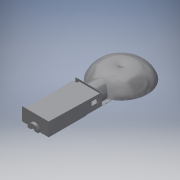
# Autodesk Inventor part: Shelter
Saved by Autodesk Inventor 2017 (Build 210142000, 142)
## iProperties
Created: 2021-04-11
Part Number: Shelter
Material: Aluminum 6061-AHC
Document SubType Name: Modeling
Designer: udays
Density: 2.7 g/cm^3
Appearance: Aluminum Cast
Author: udays
Autodesk Inventor part; units mm, degrees
ref_plane "YZ Plane" through (0, 0, 0) normal (1, 0, 0) x (0, 1, 0)
ref_plane "XZ Plane" through (0, 0, 0) normal (0, 1, 0) x (-1, 0, 0)
ref_plane "XY Plane" through (0, 0, 0) normal (0, 0, 1) x (1, 0, 0)
sketch "Sketch1" plane through (0, 0, 0) normal (0, 1, 0) x (-1, 0, 0)
  line L0 (0, 0) -> (2540, 0)
  line L1 (2540, 0) -> (2540, -5080)
  line L2 (2540, -5080) -> (0, -5080)
  line L3 (0, -5080) -> (0, 0)
  dimension "d0" = 2540
  dimension "d1" = 5080
  constraints: 8 end point, 2 parallel, 1 horizontal, 1 perpendicular
  measures "d0" distance of L1.end L2.end
  measures "d1" distance of L0.end L1.end
extrude "Extrusion1" add sketch "Sketch1" along normal blind 25.4
sketch "Sketch2" plane through (-2540, 0, 0) normal (0, 0, 1) x (1, 0, 0)
  line L0 (2540, 0) -> (0, 0) projected
  line L1 (0, 0) -> (2540, 0)
  line L2 (2540, 0) -> (2540, 1270)
  line L3 (2540, 1270) -> (0, 1270)
  line L4 (0, 1270) -> (0, 0)
  dimension "d4" = 1270
  constraints: 8 end point, 2 parallel, 1 horizontal, 1 perpendicular
  measures "d4" distance of L2.end L1.end
extrude "Extrusion2" add sketch "Sketch2" along normal blind 25.4
sketch "Sketch3" plane through (0, 25.4, 0) normal (1, 0, 0) x (0, 0, -1)
  line L0 (5080, -25.4) -> (-25.4, -25.4) projected
  line L1 (-25.4, -25.4) -> (5105.4, -25.4)
  line L2 (5105.4, -25.4) -> (5105.4, 1117.6)
  line L3 (-25.4, 1244.6) -> (-25.4, -25.4) projected
  line L4 (-25.4, -25.4) -> (-25.4, 1244.6)
  line L5 (-25.4, 1244.6) -> (5105.4, 1117.6)
  point P0 (0, -25.4)
  dimension "d8" = 1143
  dimension "d35" = 1270
  constraints: 8 end point, 1 collinear, 1 horizontal, 1 perpendicular
  measures "d8" distance of L2.end L1.end
  measures "d35" distance of L0.end L3.start
extrude "Extrusion3" add sketch "Sketch3" along normal blind 25.4
sketch "Sketch4" plane through (0, 0, -5105.4) normal (0, 0, -1) x (-1, 0, 0)
  arc A0 (2159, 0) -> (1270, 889) centre (1270, 0) ccw
  arc A1 (1270, 889) -> (381, 0) centre (1270, 0) ccw
  line L0 (2540, 1143) -> (5105.4, 1143) construction
  line L1 (2540, 0) -> (-25.4, 0) projected
  line L2 (2540, 0) -> (2540, 1143)
  line L3 (2540, 1143) -> (-25.4, 1143)
  line L4 (-25.4, 1143) -> (-25.4, 0)
  line L5 (-25.4, 0) -> (381, 0)
  line L6 (2159, 0) -> (2540, 0)
  dimension "d32" = 1143
  constraints: 12 end point, 5 point on circle, 3 horizontal, 3 parallel, 2 centre point, 2 perpendicular, 1 coincident
  measures "d32" distance of L0.start L2.start
ref_plane "Work Plane1" through (0, 0, -5130.8) normal (0, 0, -1) x (-1, 0, 0)
sketch "Sketch7" plane through (0, 0, -5130.8) normal (0, 0, -1) x (-1, 0, 0)
  line L0 (2540, 0) -> (0, 0) projected
  arc A0 (2235.2, 0) -> (1270, 965.2) centre (1270, 0) ccw
  arc A1 (1270, 965.2) -> (304.8, 0) centre (1270, 0) ccw
  line L1 (304.8, 0) -> (2235.2, 0)
  dimension "d17" = 965.2
  constraints: 4 point on circle, 2 centre point, 2 end point, 1 coincident, 1 collinear, 1 midpoint
  measures "d17" radius of A0
extrude "Extrusion6" add sketch "Sketch7" along normal blind 1536.7
extrude "Extrusion9" add sketch "Sketch4" along normal blind 25.4 contours A0 A1 L1 L4 L3 L2
sketch "Sketch12" plane through (0, 0, -5080) normal (0, 0, -1) x (-1, 0, 0)
  line L0 (2540, 0) -> (-25.4, 0) projected
  line L1 (2540, 1270) -> (2540, 25.4) projected
  line L2 (-25.4, 0) -> (2540, 0)
  line L3 (2540, 0) -> (2540, 25.4)
  line L4 (2540, 25.4) -> (-25.4, 25.4)
  line L5 (-25.4, 25.4) -> (-25.4, 0)
  point P0 (0, 0)
  constraints: 8 end point, 2 parallel, 1 horizontal, 1 perpendicular
extrude "Extrusion11" add sketch "Sketch12" along normal blind 1898.65
fillet "Fillet2" radius 39.6875 1 edges at (-1270, 889, -5130.8)
ref_plane "Work Plane4" through (0, 0, -8262.4422) normal (0, 0, -1) x (-1, 0, 0)
sketch "Sketch14" plane through (0, 0, -8262.4422) normal (0, 0, -1) x (-1, 0, 0)
  line L0 (2540, 25.4) -> (0, 25.4) projected
  line L1 (1270, 25.4) -> (3810, 25.4)
  line L2 (1270, 25.4) -> (1270, 1117.6)
  arc A0 (3810, 25.4) -> (1270, 1117.6) centre (2045.9544, -577.4432) ccw
  point P0 (0, 0)
  dimension "d48" = 2540
  dimension "d49" = 1092.2
  constraints: 4 end point, 2 point on circle, 1 centre point, 1 collinear, 1 midpoint, 1 perpendicular
  measures "d48" distance of L1.start L1.end
  measures "d49" distance of L1.start L2.end
revolve "Revolution1" add sketch "Sketch14" angle 360 about axis through (-1270, 25.4, -8262.4422) along (0, 1, 0)
sketch "Sketch16" plane through (0, 0, -5130.8) normal (0, 0, 1) x (1, 0, 0)
  line L0 (25.4, 0) -> (-2540, 0) projected
  line L1 (-1257.3, 0) -> (-1257.3, 28.575)
  arc A0 (-495.3, 28.575) -> (-1257.3, 790.575) centre (-1257.3, 28.575) ccw
  line L2 (-1257.3, 28.575) -> (-1257.3, 790.575) construction
  line L3 (-1257.3, 28.575) -> (-495.3, 28.575) construction
  line L4 (-1257.3, 28.575) -> (-495.3, 28.575) construction
  arc A1 (-1257.3, 790.575) -> (-2019.3, 28.575) centre (-1257.3, 28.575) ccw
  line L5 (-1257.3, 28.575) -> (-2019.3, 28.575) construction
  line L6 (-1257.3, 28.575) -> (-1257.3, 790.575) construction
  arc A2 (-495.3, 28.575) -> (-2019.3, 28.575) centre (-1257.3, 28.575) ccw
  line L7 (-2019.3, 28.575) -> (-495.3, 28.575)
  point P0 (0, 0)
  dimension "d51" = 28.575
  dimension "d52" = 762
  dimension "d53" = 90
  dimension "d54" = 90
  dimension "d55" = 90
  constraints: 14 end point, 7 point on circle, 3 centre point, 2 coincident, 1 concentric, 1 horizontal, 1 midpoint, 1 perpendicular, 1 vertical
  measures "d51" distance of L1.start L1.end
  measures "d52" radius of A0
  measures "d53" angle of L3 L2
  measures "d54" angle of L4 L2
  measures "d55" angle of L6 L5
extrude "Extrusion12" cut sketch "Sketch16" against normal blind 5027.6125
sketch "Sketch18" plane through (-2540, 0, 25.4) normal (0, 0, 1) x (1, 0, 0)
  arc A0 (2121.4941, 28.575) -> (419.2797, 46.1929) centre (1270, 0) ccw projected
  line L0 (1786.8174, 24.4898) -> (770.8174, 24.4898) construction
  line L1 (1786.8174, 24.4898) -> (2802.8174, 24.4898) construction
  line L2 (770.8174, 24.4898) -> (1786.8174, 24.4898)
  arc A1 (1786.8174, 24.4898) -> (770.8174, 24.4898) centre (1278.8174, 49.8239) ccw
  point P0 (2540, 0)
  point P1 (1278.8174, 532.4898)
  dimension "d62" = 1016
  dimension "d63" = 180
  constraints: 6 end point, 2 collinear, 2 point on circle, 1 centre point, 1 horizontal
  measures "d62" distance of L0.start L0.end
  measures "d63" angle of L0 L1
extrude "Extrusion13" add sketch "Sketch18" along normal blind 254
sketch "Sketch19" plane through (0, 25.4, 0) normal (0, 1, 0) x (1, 0, 0)
  line L0 (0, 5105.4) -> (0, 0) projected
  line L1 (0, 0) -> (-2540, 0) projected
  line L2 (0, 1699.357) -> (-752.9015, 1699.357)
  line L3 (-752.9015, 1699.357) -> (-752.9015, 0)
  line L4 (-752.9015, 0) -> (0, 0)
  line L5 (0, 0) -> (0, 1699.357)
  line L6 (0, 0) -> (-726.44, 0)
  line L7 (-726.44, 0) -> (-726.44, 1673.86)
  line L8 (-726.44, 1673.86) -> (0, 1673.86)
  line L9 (0, 1673.86) -> (0, 0)
  dimension "d66" = 726.44
  dimension "d67" = 1673.86
  constraints: 16 end point, 4 parallel, 2 horizontal, 2 perpendicular, 2 point on line
  measures "d66" distance of L7.end L8.end
  measures "d67" distance of L6.end L7.end
extrude "Extrusion14" add sketch "Sketch19" along normal blind 914.4 contours L0 L8 L7 L1 L3 L2
sketch "Sketch20" plane through (0, 25.4, 0) normal (0, 1, 0) x (1, 0, 0)
  line L0 (-2540, 0) -> (-2540, 5105.4) projected
  line L1 (-2540, 0) -> (-1778, 0)
  line L2 (-1778, 0) -> (-1778, 2032)
  line L3 (-1778, 2032) -> (-2540, 2032)
  line L4 (-2540, 2032) -> (-2540, 0)
  line L5 (-2540, 0) -> (-1803.4, 0)
  line L6 (-1803.4, 0) -> (-1803.4, 2006.6)
  line L7 (-1803.4, 2006.6) -> (-2540, 2006.6)
  line L8 (-2540, 2006.6) -> (-2540, 0)
  point P0 (0, 0)
  dimension "d70" = 762
  dimension "d71" = 2032
  dimension "d72" = 736.6
  dimension "d73" = 2006.6
  constraints: 16 end point, 4 parallel, 2 horizontal, 2 perpendicular
  measures "d70" distance of L3.end L2.end
  measures "d71" distance of L2.end L1.end
  measures "d72" distance of L7.end L6.end
  measures "d73" distance of L6.end L5.end
extrude "Extrusion15" add sketch "Sketch20" along normal blind 914.4 contours L0 L3 L2 L1 L6 L7
sketch "Sketch21" plane through (0, 25.4, 0) normal (0, 1, 0) x (1, 0, 0)
  line L0 (0, 5105.4) -> (0, 0) projected
  line L1 (0, 1699.2126) -> (-1016, 1699.2126)
  line L2 (-1016, 1699.2126) -> (-1016, 3604.2126)
  line L3 (-1016, 3604.2126) -> (0, 3604.2126)
  line L4 (0, 3604.2126) -> (0, 1699.2126)
  line L5 (-752.9015, 1699.357) -> (0, 1699.357) projected
  line L6 (0, 1699.357) -> (-990.6, 1699.357)
  line L7 (-990.6, 1699.357) -> (-990.6, 3578.957)
  line L8 (-990.6, 3578.957) -> (0, 3578.957)
  line L9 (0, 3578.957) -> (0, 1699.357)
  dimension "d76" = 1016
  dimension "d77" = 1905
  dimension "d78" = 990.6
  dimension "d79" = 1879.6
  constraints: 16 end point, 4 parallel, 2 horizontal, 2 perpendicular, 1 point on line
  measures "d76" distance of L2.end L3.end
  measures "d77" distance of L1.end L2.end
  measures "d78" distance of L7.end L8.end
  measures "d79" distance of L6.end L7.end
extrude "Extrusion16" add sketch "Sketch21" along normal blind 914.4 contours L0 L8 L7 L6 L5 L1 L2 L3
sketch "Sketch22" plane through (0, 25.4, 0) normal (0, 1, 0) x (1, 0, 0)
  line L0 (-780.5143, 1672.912) -> (-987.544, 1672.912)
  line L1 (-987.544, 1672.912) -> (-987.544, 1086.0023)
  line L2 (-987.544, 1086.0023) -> (-780.5143, 1086.0023)
  line L3 (-780.5143, 1086.0023) -> (-780.5143, 1672.912)
  line L4 (-752.9015, 0) -> (-752.9015, 1699.2126) projected
  line L5 (-752.9015, 1699.2126) -> (-1016, 1699.2126)
  line L6 (-1016, 1699.2126) -> (-1016, 1054.7525)
  line L7 (-1016, 1054.7525) -> (-752.9015, 1054.7525)
  line L8 (-752.9015, 1054.7525) -> (-752.9015, 1699.2126)
  line L9 (-1016, 3604.2126) -> (-1016, 1699.2126) projected
  line L10 (0, 1699.357) -> (-990.6, 1699.357) projected
  line L11 (-752.9015, 1699.2126) -> (-752.9015, 0) projected
  point P0 (0, 0)
  constraints: 16 end point, 7 parallel, 2 horizontal, 2 perpendicular, 1 collinear
extrude "Extrusion17" add sketch "Sketch22" along normal blind 914.4
sketch "Sketch23" plane through (0, 25.4, 0) normal (0, 1, 0) x (1, 0, 0)
  line L0 (-2540, -25.4) -> (-2540, 6978.65) projected
  line L1 (-2540, 2032.0093) -> (-2006.6, 2032.0093)
  line L2 (-2006.6, 2032.0093) -> (-2006.6, 3124.2093)
  line L3 (-2006.6, 3124.2093) -> (-2540, 3124.2093)
  line L4 (-2540, 3124.2093) -> (-2540, 2032.0093)
  line L5 (-2540, 2032.0093) -> (-2032, 2032.0093)
  line L6 (-2032, 2032.0093) -> (-2032, 3098.8093)
  line L7 (-2032, 3098.8093) -> (-2540, 3098.8093)
  line L8 (-2540, 3098.8093) -> (-2540, 2032.0093)
  point P0 (0, 0)
  dimension "d84" = 533.4
  dimension "d85" = 1092.2
  dimension "d86" = 508
  dimension "d87" = 1066.8
  constraints: 16 end point, 4 parallel, 2 horizontal, 2 perpendicular, 1 point on line
  measures "d84" distance of L3.end L2.end
  measures "d85" distance of L2.end L1.end
  measures "d86" distance of L7.end L6.end
  measures "d87" distance of L6.end L5.end
extrude "Extrusion18" add sketch "Sketch23" along normal blind 914.4 contours L0 L3 L2 L1 L6 L7
sketch "Sketch24" plane through (-2540, 25.4, -2006.6) normal (0, 0, 1) x (1, 0, 0)
  line L0 (0, 0) -> (762, 0) projected
  line L1 (212.9296, 0) -> (441.5296, 0)
  line L2 (441.5296, 0) -> (441.5296, 508)
  line L3 (441.5296, 508) -> (212.9296, 508)
  line L4 (212.9296, 508) -> (212.9296, 0)
  point P0 (2540, -25.4)
  dimension "d90" = 508
  dimension "d91" = 228.6
  constraints: 8 end point, 2 parallel, 1 horizontal, 1 perpendicular, 1 point on line
  measures "d90" distance of L1.end L2.end
  measures "d91" distance of L2.end L3.end
extrude "Extrusion19" cut sketch "Sketch24" against normal blind 914.4
sketch "Sketch25" plane through (-1803.4, 25.4, -2006.6) normal (-1, 0, 0) x (0, 0, 1)
  line L0 (2006.6, 0) -> (0, 0) projected
  line L1 (208.6355, 0) -> (437.2355, 0)
  line L2 (437.2355, 0) -> (437.2355, 508)
  line L3 (437.2355, 508) -> (208.6355, 508)
  line L4 (208.6355, 508) -> (208.6355, 0)
  point P0 (2006.6, -25.4)
  dimension "d94" = 228.6
  dimension "d95" = 508
  constraints: 8 end point, 2 parallel, 1 horizontal, 1 perpendicular, 1 point on line
  measures "d94" distance of L3.end L2.end
  measures "d95" distance of L2.end L1.end
extrude "Extrusion20" cut sketch "Sketch25" against normal blind 254
sketch "Sketch26" plane through (-1016, 25.4, -3604.2126) normal (-1, 0, 0) x (0, 0, 1)
  line L0 (25.2556, 0) -> (1904.8556, 0) projected
  line L1 (109.9537, 0) -> (338.5537, 0)
  line L2 (338.5537, 0) -> (338.5537, 508)
  line L3 (338.5537, 508) -> (109.9537, 508)
  line L4 (109.9537, 508) -> (109.9537, 0)
  point P0 (3604.2126, -25.4)
  dimension "d98" = 228.6
  dimension "d99" = 508
  constraints: 8 end point, 2 parallel, 1 horizontal, 1 perpendicular, 1 point on line
  measures "d98" distance of L3.end L2.end
  measures "d99" distance of L2.end L1.end
extrude "Extrusion21" cut sketch "Sketch26" against normal blind 254
sketch "Sketch27" plane through (-1016, 25.4, -3604.2126) normal (-1, 0, 0) x (0, 0, 1)
  line L0 (2549.4601, 0) -> (338.5537, 0) projected
  line L1 (2487.3786, 0) -> (2030.1786, 0)
  line L2 (2030.1786, 0) -> (2030.1786, 508)
  line L3 (2030.1786, 508) -> (2487.3786, 508)
  line L4 (2487.3786, 508) -> (2487.3786, 0)
  point P0 (3604.2126, -25.4)
  dimension "d102" = 457.2
  dimension "d103" = 508
  constraints: 8 end point, 2 parallel, 1 horizontal, 1 perpendicular, 1 point on line
  measures "d102" distance of L2.end L3.end
  measures "d103" distance of L1.end L2.end
extrude "Extrusion22" cut sketch "Sketch27" against normal blind 127
sketch "Sketch28" plane through (-726.44, 25.4, -1673.86) normal (0, 0, 1) x (1, 0, 0)
  line L0 (726.44, 0) -> (0, 0) projected
  line L1 (133.4076, 0) -> (590.6076, 0)
  line L2 (590.6076, 0) -> (590.6076, 508)
  line L3 (590.6076, 508) -> (133.4076, 508)
  line L4 (133.4076, 508) -> (133.4076, 0)
  point P0 (726.44, -25.4)
  dimension "d106" = 457.2
  dimension "d107" = 508
  constraints: 8 end point, 2 parallel, 1 horizontal, 1 perpendicular, 1 point on line
  measures "d106" distance of L3.end L2.end
  measures "d107" distance of L2.end L1.end
extrude "Extrusion23" cut sketch "Sketch28" against normal blind 127
sketch "Sketch29" plane through (0, 25.4, 0) normal (-1, 0, 0) x (0, 0, 1)
  line L0 (-4898.6971, 841.0224) -> (-4136.6971, 841.0224)
  line L1 (-4136.6971, 841.0224) -> (-4136.6971, 460.0224)
  line L2 (-4136.6971, 460.0224) -> (-4898.6971, 460.0224)
  line L3 (-4898.6971, 460.0224) -> (-4898.6971, 841.0224)
  point P0 (0, -25.4)
  dimension "d110" = 762
  dimension "d111" = 381
  constraints: 8 end point, 2 parallel, 1 horizontal, 1 perpendicular
  measures "d110" distance of L1.end L2.end
  measures "d111" distance of L0.end L1.end
extrude "Extrusion24" cut sketch "Sketch29" against normal blind 127
sketch "Sketch30" plane through (0, 0, -5105.4) normal (0, 0, 1) x (1, 0, 0)
  line L0 (-2540, 1143) -> (25.4, 1143) projected
  line L1 (-2484.6308, 22.8109) -> (-2281.4308, 22.8109)
  line L2 (-2281.4308, 22.8109) -> (-2281.4308, 1143)
  line L3 (-2281.4308, 1143) -> (-2484.6308, 1143)
  line L4 (-2484.6308, 1143) -> (-2484.6308, 22.8109)
  point P0 (0, 0)
  dimension "d114" = 203.2
  constraints: 8 end point, 2 parallel, 1 horizontal, 1 perpendicular, 1 point on line
  measures "d114" distance of L3.end L2.end
extrude "Extrusion25" add sketch "Sketch30" along normal blind 25.4
sketch "Sketch31" plane through (0, 939.8, 0) normal (0, 1, 0) x (1, 0, 0)
  line L0 (-726.44, 0) -> (0, 0) projected
  line L1 (0, 0) -> (-2540, 0)
  line L2 (-2540, 0) -> (-2540, 5105.4)
  line L3 (-2540, 5105.4) -> (0, 5105.4)
  line L4 (0, 5105.4) -> (0, 0)
  dimension "d117" = 2540
  dimension "d118" = 5105.4
  constraints: 8 end point, 2 parallel, 1 horizontal, 1 perpendicular
  measures "d117" distance of L2.end L3.end
  measures "d118" distance of L1.end L2.end
extrude "Extrusion26" add sketch "Sketch31" along normal blind 25.4
sketch "Sketch32" plane through (0, 965.2, 0) normal (0, 1, 0) x (1, 0, 0)
  line L0 (0, 5105.4) -> (-2281.4308, 5105.4) projected
  line L1 (-2172.3199, 5105.4) -> (-2172.3199, 4891.6778)
  line L2 (-2172.3199, 4891.6778) -> (-2540, 4891.6778)
  line L3 (-2540, 5105.4) -> (-2540, 0) projected
  line L4 (-2540, 4891.6778) -> (-2540, 5105.4)
  line L5 (-2540, -25.4) -> (-2540, 6978.65) projected
  line L6 (-2540, 5105.4) -> (-2484.6308, 5105.4) projected
  line L7 (-2484.6308, 5105.4) -> (-2484.6308, 5080)
  line L8 (-2281.4308, 5080) -> (-2484.6308, 5080) projected
  line L9 (-2484.6308, 5080) -> (-2281.4308, 5080)
  line L10 (-2281.4308, 5080) -> (-2281.4308, 5105.4)
  line L11 (-2281.4308, 5105.4) -> (-2172.3199, 5105.4)
  point P0 (0, 0)
  constraints: 14 end point, 3 perpendicular, 3 point on line, 2 vertical, 1 collinear
extrude "Extrusion27" cut sketch "Sketch32" against normal blind 25.4
sketch "Sketch33" plane through (-2540, 0, 279.4) normal (0, 0, 1) x (1, 0, 0)
  line L0 (418.4053, 25.4) -> (2121.5947, 25.4) projected
  line L1 (1107.9555, 25.4) -> (1419.1055, 25.4)
  line L2 (1419.1055, 25.4) -> (1419.1055, 444.5)
  line L3 (1419.1055, 444.5) -> (1107.9555, 444.5)
  line L4 (1107.9555, 444.5) -> (1107.9555, 25.4)
  point P0 (2540, 0)
  dimension "d123" = 311.15
  dimension "d124" = 419.1
  constraints: 8 end point, 2 parallel, 1 horizontal, 1 perpendicular, 1 point on line
  measures "d123" distance of L3.end L2.end
  measures "d124" distance of L2.end L1.end
extrude "Extrusion28" cut sketch "Sketch33" against normal blind 127
sketch "Sketch35" plane through (0, 0, 0) normal (0, -1, 0) x (1, 0, 0)
  line L0 (-1778, -2032) -> (-2540, -2032) projected
  line L1 (-1803.4, 0) -> (-1778, 0)
  line L2 (-1778, 0) -> (-1778, -2032)
  line L3 (-1778, -2032) -> (-1803.4, -2032)
  line L4 (-1803.4, -2032) -> (-1803.4, 0)
  line L5 (-2327.0704, -2006.6) -> (-2540, -2006.6) projected
  line L6 (-1803.4, -2032) -> (-2540, -2032)
  line L7 (-2540, -2032) -> (-2540, -2006.6)
  line L8 (-2540, -2006.6) -> (-1803.4, -2006.6)
  line L9 (-1803.4, -2006.6) -> (-1803.4, -2032)
  line L10 (-2006.6, -3124.2093) -> (-2006.6, -2032.0093) projected
  line L11 (-2540, -3125.3293) -> (-2006.6, -3125.3293)
  line L12 (-2006.6, -3125.3293) -> (-2006.6, -3096.9647)
  line L13 (-2006.6, -3096.9647) -> (-2540, -3096.9647)
  line L14 (-2540, -3096.9647) -> (-2540, -3125.3293)
  line L15 (-2032, -3098.8093) -> (-2540, -3098.8093) projected
  line L16 (-2054.3384, -3098.8093) -> (-2006.6, -3098.8093)
  line L17 (-2006.6, -3098.8093) -> (-2006.6, -2032)
  line L18 (-2006.6, -2032) -> (-2054.3384, -2032)
  line L19 (-2054.3384, -2032) -> (-2054.3384, -3098.8093)
  line L20 (-1016, -3604.2126) -> (-1016, -1054.7525) projected
  line L21 (-1778, -1792.9013) -> (-1016, -1792.9013)
  line L22 (-1016, -1792.9013) -> (-1016, -1723.8766)
  line L23 (-1016, -1723.8766) -> (-1778, -1723.8766)
  line L24 (-1778, -1723.8766) -> (-1778, -1792.9013)
  line L25 (0, -1699.357) -> (-990.6, -1699.357) projected
  line L26 (0, -3578.957) -> (0, -1699.357) projected
  line L27 (-969.1357, -1699.357) -> (0, -1699.357)
  line L28 (0, -1699.357) -> (0, -3578.957)
  line L29 (0, -3578.957) -> (-969.1357, -3578.957)
  line L30 (-969.1357, -3578.957) -> (-969.1357, -1699.357)
  line L31 (25.4, -5105.4) -> (25.4, 25.4) projected
  line L32 (-1016, -3602.8805) -> (25.4, -3602.8805)
  line L33 (25.4, -3602.8805) -> (25.4, -1674.0255)
  line L34 (25.4, -1674.0255) -> (-1016, -1674.0255)
  line L35 (-1016, -1674.0255) -> (-1016, -3602.8805)
  line L36 (-726.44, 0) -> (-726.44, -1673.86) projected
  line L37 (0, 0) -> (0, 25.4) projected
  line L38 (-726.44, -1673.86) -> (0, -1673.86)
  line L39 (0, -1673.86) -> (0, 0)
  line L40 (0, 0) -> (-726.44, 0)
  line L41 (-726.44, 0) -> (-726.44, -1673.86)
  line L42 (-780.5143, -1672.912) -> (25.4, -1672.912)
  line L43 (25.4, -1672.912) -> (25.4, 25.4)
  line L44 (25.4, 25.4) -> (-780.5143, 25.4)
  line L45 (-780.5143, 25.4) -> (-780.5143, -1672.912)
  line L46 (-1120.8945, 152.4) -> (-1432.0445, 152.4) projected
  line L47 (-1310.4242, 152.4) -> (-1241.3995, 152.4)
  line L48 (-1241.3995, 152.4) -> (-1241.3995, -1723.8766)
  line L49 (-1241.3995, -1723.8766) -> (-1310.4242, -1723.8766)
  line L50 (-1310.4242, -1723.8766) -> (-1310.4242, 152.4)
  line L51 (-2172.3199, -5105.4) -> (0, -5105.4) projected
  line L52 (-1538.8101, -1792.9013) -> (-1656.4809, -1792.9013)
  line L53 (-1656.4809, -1792.9013) -> (-1656.4809, -5105.4)
  line L54 (-1656.4809, -5105.4) -> (-1538.8101, -5105.4)
  line L55 (-1538.8101, -5105.4) -> (-1538.8101, -1792.9013)
  line L56 (-2234.8657, -5130.8) -> (-2540, -5130.8) projected
  line L57 (-2540, -5130.8) -> (25.4, -5130.8)
  line L58 (25.4, -5130.8) -> (25.4, -5105.4)
  line L59 (25.4, -5105.4) -> (-2540, -5105.4)
  line L60 (-2540, -5105.4) -> (-2540, -5130.8)
  line L61 (-2234.8657, -5130.8) -> (-305.1343, -5130.8) projected
  line L62 (-2540, -6978.65) -> (25.4, -6978.65) projected
  line L63 (-1049.1193, -5130.8) -> (-997.3583, -5130.8)
  line L64 (-997.3583, -5130.8) -> (-997.3583, -6978.65)
  line L65 (-997.3583, -6978.65) -> (-1049.1193, -6978.65)
  line L66 (-1049.1193, -6978.65) -> (-1049.1193, -5130.8)
  line L67 (-2006.6, -5130.8) -> (-1960.5053, -5130.8)
  line L68 (-1960.5053, -5130.8) -> (-1960.5053, -6978.65)
  line L69 (-1960.5053, -6978.65) -> (-2006.6, -6978.65)
  line L70 (-2006.6, -6978.65) -> (-2006.6, -5130.8)
  line L71 (-1049.1193, -6518.5676) -> (-1960.5053, -6518.5676)
  line L72 (-1960.5053, -6518.5676) -> (-1960.5053, -6486.1043)
  line L73 (-1960.5053, -6486.1043) -> (-1049.1193, -6486.1043)
  line L74 (-1049.1193, -6486.1043) -> (-1049.1193, -6518.5676)
  line L75 (25.4, -5130.8) -> (25.4, -6077.5992) projected
  line L76 (-997.3583, -5565.3264) -> (25.4, -5565.3264)
  line L77 (25.4, -5565.3264) -> (25.4, -5604.1996)
  line L78 (25.4, -5604.1996) -> (-997.3583, -5604.1996)
  line L79 (-997.3583, -5604.1996) -> (-997.3583, -5565.3264)
  constraints: 128 end point, 32 parallel, 24 point on line, 16 horizontal, 16 perpendicular, 1 midpoint
extrude "Extrusion29" add sketch "Sketch35" along normal blind 50.8 contours L0 L4 L1 L2 | L0 L7 L5 L8 L4 | L2 L23 L20 L21 | L17 L10 L13 L19 L0 | L21 L55 L51 L53 | L50 L46 L48 L23 | L19 L15 L14 L13 | L13 L10 L16 L15 L19 | L20 L34 L31 L32 | L15 L16 L10 L12 L11 L14 | L75 L78 L64 L76 | L57 L68 L62 L70 | L64 L62 L66 L57 | L73 L66 L71 L68 | L42 L39 L37 L44 L31 | L42 L36 L40 L39 | L37 L40 L36 L42 L45 L44
body "Solid1"
